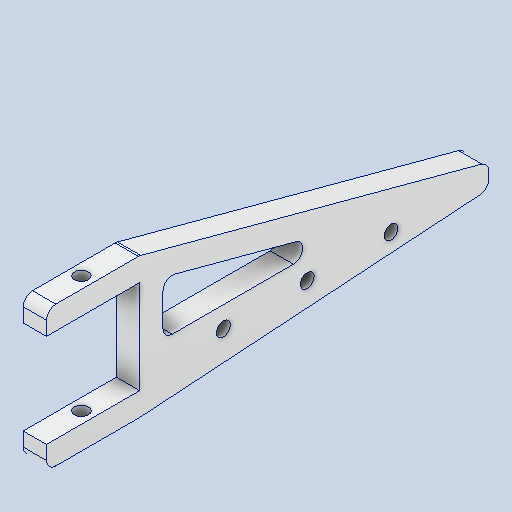
# Autodesk Inventor part: base_weel-v2-Plate-7
Saved by Autodesk Inventor 2025.2 (Build 292293000, 293)
## iProperties
Created: 2025-01-14
Part Number: base_weel-v2-Plate-7
Material: アルミニウム 6061
Document SubType Name: Modeling
Designer: haruy
Density: 2.7 g/cm^3
Appearance: アルミニウム - フラット
Author: haruy
Autodesk Inventor part; units mm, degrees
ref_plane "YZ Plane" through (0, 0, 0) normal (1, 0, 0) x (0, 1, 0)
ref_plane "XZ Plane" through (0, 0, 0) normal (0, 1, 0) x (-1, 0, 0)
ref_plane "XY Plane" through (0, 0, 0) normal (0, 0, 1) x (1, 0, 0)
sketch "スケッチ1" plane through (0, 0, 0) normal (1, 0, 0) x (0, 1, 0)
  line L0 (0, 0) -> (20.1, 0)
  line L1 (20.1, 0) -> (20.1, -20)
  line L2 (20.1, -20) -> (0, -20)
  line L3 (0, -20) -> (0, 0)
  line L4 (0, -20) -> (5, -20)
  line L5 (5, -20) -> (5, -95)
  line L6 (5, -95) -> (0, -95)
  line L7 (0, -95) -> (0, -20)
  circle A0 centre (2.5, -38) radius 1.5
  circle A1 centre (2.5, -56) radius 1.5
  circle A2 centre (2.5, -74) radius 1.5
  line L8 (20.1, 0) -> (25.1, 0)
  line L9 (25.1, 0) -> (25.1, -20)
  line L10 (25.1, -20) -> (20.1, -20)
  line L11 (20.1, -20) -> (20.1, 0)
  line L12 (0, 0) -> (-5, 0)
  line L13 (-5, 0) -> (-5, -20)
  line L14 (-5, -20) -> (0, -20)
  line L15 (0, -20) -> (0, 0)
  line L16 (25.1, -20) -> (5, -95)
  line L17 (-5, -20) -> (0, -95)
  line L18 (25.1, -25) -> (15.1, -25)
  line L19 (15.1, -25) -> (15.1, 0.1)
  line L20 (0, -25) -> (25.1, -25)
  line L21 (25.1, -25) -> (25.1, 0.1)
  line L22 (20.2704, -18.7057) -> (0.1704, -93.7057)
  line L23 (7, -95) -> (7, -18)
  line L24 (7, -18) -> (0, -18)
  point P0 (7, -25)
  point P1 (18.5836, -25)
  point P2 (7, -68.2222)
  dimension "d0" = 20.1
  dimension "d1" = 20
  dimension "d2" = 5
  dimension "d3" = 75
  dimension "d4" = 3
  dimension "d5" = 3
  dimension "d6" = 3
  dimension "d7" = 2.5
  dimension "d8" = 2.5
  dimension "d9" = 2.5
  dimension "d10" = 18
  dimension "d11" = 18
  dimension "d12" = 18
  dimension "d13" = 5
  dimension "d14" = 5
  dimension "d15" = 0
  dimension "d16" = 0
  dimension "d17" = 5
  dimension "d18" = 5
  dimension "d19" = 5
  dimension "d20" = 2
  constraints: 50 end point, 9 parallel, 5 perpendicular, 4 horizontal, 3 centre point, 3 other
  measures "d0" distance of L1.end L2.end
  measures "d1" distance of L0.end L1.end
  measures "d2" distance of L5.end L6.end
  measures "d3" distance between parallel lines of L6 L2
  measures "d4" diameter of A0
  measures "d5" diameter of A1
  measures "d6" diameter of A2
  measures "d7" distance from line of A0.centre L7
  measures "d8" distance from line of A1.centre L7
  measures "d9" distance from line of A2.centre L7
  measures "d10" distance from line of A0.centre L2
  measures "d11" distance of A1.centre A0.centre
  measures "d12" distance of A2.centre A1.centre
  measures "d13" distance of L9.end L10.end
  measures "d14" distance of L14.end L13.end
  measures "d15" distance between parallel lines of L10 L2
  measures "d16" distance between parallel lines of L4 L14
  measures "d17" distance between parallel lines of L10 L18
  measures "d18" distance between parallel lines of L2 L20
  measures "d19" distance between parallel lines of L16 L22
  measures "d20" distance between parallel lines of L5 L23
extrude "押し出し1" add sketch "スケッチ1" against normal blind 5 contours L3 L14 L13 L12 | L8 L9 L10 L1 | L19 L20 L23 L2 | L2 L22 L18 L19 | L2 L5 L20 L7 | L7 L17 L14 | L2 L10 L16 L18 L22 | L23 L20 L5 L2 | L20 L5 L6 L7 | L18 L16 L23 L22 | L23 L22 L5 L20 | L5 L22 L23 L16
fillet "フィレット1" radius 2 9 edges at (-2.5, 7, -25) (-2.5, 18.5836, -25) (-2.5, 7, -68.2222) (-2.5, 25.1, 0) (-2.5, 25.1, -20) (-2.5, -5, 0) (-2.5, -5, -20) (-2.5, 0, -95) (-2.5, 5, -95)
sketch "スケッチ2" plane through (0, 25.1, 0) normal (0, 1, 0) x (1, 0, 0)
  line L0 (0, 0) -> (-5, 0) projected
  line L1 (-5, 2) -> (-5, 19.7366) projected
  point P0 (-2.5, 10)
  point P1 (-5, 20.1)
  dimension "d24" = 10
  dimension "d25" = 2.5
  measures "d24" distance from line of L0 point (-2.5, 10)
  measures "d25" distance from line of point (-2.5, 10) L1
hole "穴1" at (-2.5, 25.1, -10) direction (0, -1, 0) diameter 3 end through all
equation "\"d8\" = d7"
equation "\"d9\" = d7"
equation "\"d11\" = d10"
equation "\"d12\" = d10"
